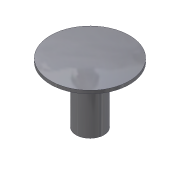
# Autodesk Inventor part: BUSS-RIVET
Saved by Autodesk Inventor 2014 (Build 180170000, 170)
## iProperties
Shininess: 64.0
Length Units: 11272
Angle Units: 11279
Time Units: 11290
Mass Units: 11286
Length Display Precision: 3
Angle Display Precision: 2
Compacted: True
Part Number: BUSS-RIVET
Document SubType Name: Modeling
Created: 2003-01-10
Designer: geyerm
Density: 1 g/cm^3
Material: Generic
Appearance: Metal-Steel (Polished)
Density: 0.0
Volumn: 0.0
Area: 0.0
PropertySet Name: Model Information
Control State: 0
Master: False
Checked Out: False
Author: Autodesk
Autodesk Inventor part; units mm, degrees
ref_plane "YZ Plane" through (0, 0, 0) normal (1, 0, 0) x (0, 1, 0)
ref_plane "XZ Plane" through (0, 0, 0) normal (0, 1, 0) x (-1, 0, 0)
ref_plane "XY Plane" through (0, 0, 0) normal (0, 0, 1) x (1, 0, 0)
sketch "Sketch1" plane through (0, 0, 0) normal (0, 0, 1) x (1, 0, 0)
  line L0 (14.2769, 21.321) -> (14.2769, 22.083) projected
  line L1 (19.431, 22.083) -> (19.431, 21.321) projected
  line L2 (19.0774, 21.7863) -> (19.0774, 21.6106)
  line L3 (16.8647, 21.6106) -> (14.6519, 21.6106)
  line L4 (14.6519, 21.6106) -> (14.6519, 21.7863)
  arc A0 (16.8647, 22.04) -> (14.6519, 21.7863) centre (16.8647, 12.2634) ccw
  line L5 (16.8647, 21.6106) -> (16.8647, 22.04)
  constraints: 8 end point, 2 parallel, 2 point on circle, 1 centre point
revolve "Revolution1" add sketch "Sketch1" angle 360 about axis through (16.8647, 21.6106, 0) along (0, 1, 0)
sketch "Sketch2" plane through (16.8647, 21.6106, 0) normal (0, -1, 0) x (1, 0, 0)
  circle A0 centre (0, 0) radius 2.2127 projected
  circle A1 centre (0, 0) radius 0.7773
  constraints: 1 centre point, 1 coincident, 1 concentric
extrude "Extrusion1" add sketch "Sketch2" along normal blind 3.175 contours A1
body "Solid1"
